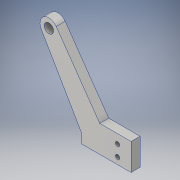
# Autodesk Inventor part: Mass 1 Insert
Saved by Autodesk Inventor 2016 (Build 200138000, 138)
## iProperties
Created: 2015-06-03
Part Number: Mass 1 Insert
Material: Aluminum 6061
Document SubType Name: Modeling
Designer: Dennis
Density: 2.7 g/cm^3
Appearance: Aluminum - Flat
Mass: 18.0158 g
Surface Area: 35.5723 cm^2
Volume: 6.67254 cm^3
Author: Dennis
Autodesk Inventor part; units mm, degrees
ref_plane "YZ Plane" through (0, 0, 0) normal (1, 0, 0) x (0, 1, 0)
ref_plane "XZ Plane" through (0, 0, 0) normal (0, 1, 0) x (-1, 0, 0)
ref_plane "XY Plane" through (0, 0, 0) normal (0, 0, 1) x (1, 0, 0)
sketch "Sketch1" plane through (0, 0, 0) normal (0, 0, 1) x (1, 0, 0)
  line L0 (0, 0) -> (-34.925, 0)
  line L1 (-34.925, 0) -> (-34.925, 6.35)
  line L2 (-22.225, 19.05) -> (0, 19.05)
  line L3 (0, 19.05) -> (0, 0)
  circle A0 centre (-58.2419, 59.436) radius 3.302
  line L4 (-58.2419, 59.436) -> (-34.925, 19.05) construction
  line L5 (-53.0395, 63.0771) -> (-22.225, 19.05)
  line L6 (-34.925, 6.35) -> (-63.7411, 56.261)
  line L7 (-34.925, 6.35) -> (-34.925, 19.05) construction
  line L8 (-22.225, 19.05) -> (-34.925, 19.05) construction
  circle A1 centre (-9.525, 12.7) radius 1.5
  circle A2 centre (-9.525, 4.7625) radius 1.5
  arc A3 (-53.0395, 63.0771) -> (-63.7411, 56.261) centre (-58.2419, 59.436) ccw
  dimension "d0" = 34.925
  dimension "d1" = 19.05
  dimension "d2" = 6.604
  dimension "d3" = 150
  dimension "d4" = 40.386
  dimension "d16" = 25.4
  dimension "d17" = 6.35
  dimension "d18" = 7.9375
  dimension "d19" = 25.4
  dimension "d20" = 3
  dimension "d21" = 3
  dimension "d22" = 12.7
  dimension "d23" = 12.7
  dimension "d24" = 12.7
  constraints: 19 end point, 4 centre point, 2 parallel, 2 perpendicular, 2 point on circle, 2 tangent, 1 coincident, 1 collinear, 1 horizontal
  measures "d0" distance of L0.start L0.end
  measures "d1" distance of L2.end L0.start
  measures "d2" diameter of A0
  measures "d3" angle of L4 L1
  measures "d4" vertical distance of L4.start L4.end
  measures "d16" distance from line of A2.centre L1
  measures "d17" distance from line of A1.centre L2
  measures "d18" distance of A2.centre A1.centre
  measures "d19" distance from line of L1 A1.centre
  measures "d20" diameter of A1
  measures "d21" diameter of A2
  measures "d22" distance of L2.start L4.end
  measures "d23" distance of L1.end L4.end
  measures "d24" diameter of A3
extrude "Extrusion1" add sketch "Sketch1" along normal blind 6.35
thread "Thread1" size "M3x0.5" class "6H" standard "ANSI Metric M Profile" full length
thread "Thread2" size "5-40 UNC" class "2B" standard "ANSI Unified Screw Threads" full length
body "Solid1"
